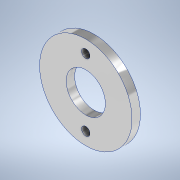
# Autodesk Inventor part: Arandela Rodamiento Lineal
Saved by Autodesk Inventor 2020 (Build 240168000, 168)
## iProperties
Created: 2020-05-17
Part Number: Arandela Rodamiento Lineal
Material: Aluminum 6061
Document SubType Name: Modeling
Designer: Dante
Density: 2.7 g/cm^3
Appearance: Aluminum - Flat
Mass: 5.56651 g
Surface Area: 18.7396 cm^2
Volume: 2.06167 cm^3
Author: Dante
Autodesk Inventor part; units mm, degrees
ref_plane "YZ Plane" through (0, 0, 0) normal (1, 0, 0) x (0, 1, 0)
ref_plane "XZ Plane" through (0, 0, 0) normal (0, 1, 0) x (-1, 0, 0)
ref_plane "XY Plane" through (0, 0, 0) normal (0, 0, 1) x (1, 0, 0)
sketch "Sketch1" plane through (0, 0, 0) normal (0, 0, 1) x (1, 0, 0)
  circle A0 centre (41.6247, 32.3639) radius 7
  circle A1 centre (41.6247, 32.3639) radius 16.5
  circle A2 centre (41.6247, 44.3639) radius 1.5
  circle A3 centre (41.6247, 20.3639) radius 1.5
  dimension "d0" = 14
  dimension "d5" = 3
  dimension "d7" = 3
  dimension "d19" = 33
  dimension "d24" = 0
  dimension "d25" = 0
  dimension "d26" = 24
  dimension "d30" = 12
  constraints: 4 centre point, 1 coincident
  measures "d0" diameter of A0
  measures "d5" diameter of A2
  measures "d7" diameter of A3
  measures "d19" diameter of A1
  measures "d24" horizontal distance of A2.centre A0.centre
  measures "d25" horizontal distance of A3.centre A0.centre
  measures "d26" distance of A2.centre A3.centre
  measures "d30" distance of A3.centre A0.centre
extrude "Extrusion1" add sketch "Sketch1" along normal blind 3
body "Solid1"
